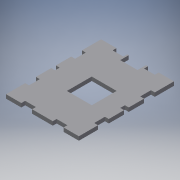
# Autodesk Inventor part: Part8
Saved by Autodesk Inventor 2018 (Build 220112000, 112)
## iProperties
Created: 2018-05-22
Part Number: Part8
Material: Generic
Document SubType Name: Modeling
Designer: Administrator
Density: 1 g/cm^3
Appearance: Default
Author: Administrator
Autodesk Inventor part; units mm, degrees
ref_plane "YZ Plane" through (0, 0, 0) normal (1, 0, 0) x (0, 1, 0)
ref_plane "XZ Plane" through (0, 0, 0) normal (0, 1, 0) x (-1, 0, 0)
ref_plane "XY Plane" through (0, 0, 0) normal (0, 0, 1) x (1, 0, 0)
sketch "Sketch1" plane through (0, 0, 0) normal (0, 1, 0) x (-1, 0, 0)
  line L0 (-11.8108, -30.2381) -> (15.1767, -30.2381)
  line L1 (15.1767, -30.2381) -> (15.1767, 5.9569)
  line L2 (15.1767, 5.9569) -> (-11.8108, 5.9569)
  line L3 (-11.8108, 5.9569) -> (-11.8108, -30.2381)
  line L4 (-11.8108, -30.2381) -> (-14.9858, -30.2381)
  line L5 (-14.9858, -30.2381) -> (-14.9858, -17.5381)
  line L6 (-14.9858, -17.5381) -> (-11.8108, -17.5381)
  line L7 (-11.8108, -17.5381) -> (-11.8108, -30.2381)
  line L8 (-11.8108, -8.6481) -> (-14.9858, -8.6481)
  line L9 (-14.9858, -8.6481) -> (-14.9858, 4.0519)
  line L10 (-14.9858, 4.0519) -> (-11.8108, 4.0519)
  line L11 (-11.8108, 4.0519) -> (-11.8108, -8.6481)
  line L12 (-14.9858, -30.2381) -> (-2.2858, -30.2381)
  line L13 (-2.2858, -30.2381) -> (-2.2858, -33.4131)
  line L14 (-2.2858, -33.4131) -> (-14.9858, -33.4131)
  line L15 (-14.9858, -33.4131) -> (-14.9858, -30.2381)
  line L16 (15.1767, -30.2381) -> (6.6042, -30.2381)
  line L17 (6.6042, -30.2381) -> (6.6042, -33.4131)
  line L18 (6.6042, -33.4131) -> (15.1767, -33.4131)
  line L19 (15.1767, -33.4131) -> (15.1767, -30.2381)
  point P0 (0, 0)
  dimension "d0" = 26.9875
  dimension "d1" = 36.195
  dimension "d5" = 3.175
  dimension "d6" = 12.7
  dimension "d7" = 8.89
  dimension "d8" = 12.7
  dimension "d10" = 12.7
  dimension "d11" = 8.89
  constraints: 40 end point, 10 parallel, 5 horizontal, 5 perpendicular, 1 point on line
  measures "d0" distance between parallel lines of L1 L3
  measures "d1" distance between parallel lines of L2 L0
  measures "d5" distance between parallel lines of L5 L3
  measures "d6" distance between parallel lines of L4 L6
  measures "d7" distance between parallel lines of L8 L6
  measures "d8" distance between parallel lines of L10 L8
  measures "d10" distance between parallel lines of L15 L13
  measures "d11" distance between parallel lines of L13 L17
extrude "Extrusion1" add sketch "Sketch1" along normal blind 3.175
mirror "Mirror1" about plane through (-15.1767, 0, 5.9569) normal (0, 0, 1) of "Extrusion1"
mirror "Mirror2" about plane through (-15.1767, 0, -33.4131) normal (-1, 0, 0) of "Extrusion1", "Mirror1"
sketch "Sketch2" plane through (0, 3.175, 0) normal (0, 1, 0) x (1, 0, 0)
  line L0 (-1.9052, 2.8061) -> (-22.4792, 2.8061)
  line L1 (-22.4792, 2.8061) -> (-22.4792, -17.7679)
  line L2 (-22.4792, -17.7679) -> (-1.9052, -17.7679)
  line L3 (-1.9052, -17.7679) -> (-1.9052, 2.8061)
  line L4 (14.9858, -7.8619) -> (14.9858, -20.5619) projected
  line L5 (-45.3392, -7.8619) -> (-45.3392, -20.5619) projected
  line L6 (-23.7492, -45.3269) -> (-6.6042, -45.3269) projected
  line L7 (-6.6042, 33.4131) -> (-23.7492, 33.4131) projected
  line L8 (-22.4792, 26.4281) -> (-8.2552, 26.4281)
  line L9 (-8.2552, 26.4281) -> (-8.2552, 33.4131)
  line L10 (-8.2552, 33.4131) -> (-22.4792, 33.4131)
  line L11 (-22.4792, 33.4131) -> (-22.4792, 26.4281)
  point P0 (0, 0)
  dimension "d14" = 20.574
  dimension "d15" = 16.891
  dimension "d16" = 22.86
  dimension "d17" = 27.559
  dimension "d18" = 20.574
  dimension "d19" = 14.224
  dimension "d20" = 6.985
  constraints: 16 end point, 4 parallel, 2 horizontal, 2 perpendicular, 1 point on line
  measures "d14" distance between parallel lines of L3 L1
  measures "d15" distance between parallel lines of L4 L3
  measures "d16" distance between parallel lines of L5 L1
  measures "d17" distance between parallel lines of L6 L2
  measures "d18" distance between parallel lines of L2 L0
  measures "d19" distance between parallel lines of L9 L11
  measures "d20" distance between parallel lines of L7 L8
extrude "Extrusion2" cut sketch "Sketch2" against normal blind 3.175
body "Solid1"
